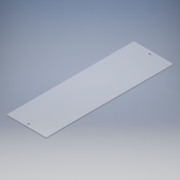
# Autodesk Inventor part: FrontCagePanelRemovable
Saved by Autodesk Inventor 2018 (Build 220112000, 112)
## iProperties
Created: 2013-02-21
Part Number: FrontCagePanelRemovable
Material: PVC-U
Document SubType Name: Modeling
Designer: Neef
Mass: 592.561 g
Surface Area: 1495.34 cm^2
Volume: 423.258 cm^3
Density: 1.29 g/cm^3
Appearance: Smooth - White
Author: Neef
Autodesk Inventor part; units mm, degrees
ref_plane "YZ Plane" through (0, 0, 0) normal (1, 0, 0) x (0, 1, 0)
ref_plane "XZ Plane" through (0, 0, 0) normal (0, 1, 0) x (-1, 0, 0)
ref_plane "XY Plane" through (0, 0, 0) normal (0, 0, 1) x (1, 0, 0)
sketch "Skizze1" plane through (0, 0, 0) normal (0, 0, 1) x (1, 0, 0)
  line L0 (0, 406) -> (0, -406) projected
  line L1 (-126, 0) -> (126, 0) projected
  line L2 (-90, -290) -> (90, -290)
  line L3 (90, -290) -> (90, 290)
  line L4 (90, 290) -> (-90, 290)
  line L5 (-90, 290) -> (-90, -290)
  point P0 (0, 0)
  point P1 (0, -290)
  point P2 (-90, 0)
  dimension "d0" = 580
  dimension "d1" = 180
  constraints: 8 end point, 2 midpoint, 2 parallel, 2 point on line, 1 horizontal, 1 perpendicular
  measures "d0" distance of L4.end L2.start
  measures "d1" distance of L2.start L2.end
extrude "Extrusion1" add sketch "Skizze1" along normal blind 6
sketch "Sketch4" plane through (0, 0, 6) normal (0, 0, 1) x (1, 0, 0)
  circle A0 centre (-3.75, -276) radius 3.825
  line L0 (90, 290) -> (90, -290) projected
  line L1 (90, -290) -> (-90, -290) projected
  circle A1 centre (-3.75, 276) radius 3.825
  line L2 (-90, 290) -> (90, 290) projected
  point P0 (0, 0)
  dimension "d11" = 7.65
  dimension "d12" = 93.75
  dimension "d13" = 14
  dimension "d14" = 7.65
  dimension "d15" = 14
  dimension "d16" = 93.75
  constraints: 2 centre point
  measures "d11" diameter of A0
  measures "d12" distance from line of L0 A0.centre
  measures "d13" distance from line of L1 A0.centre
  measures "d14" diameter of A1
  measures "d15" distance from line of L2 A1.centre
  measures "d16" distance from line of L0 A1.centre
extrude "Extrusion3" cut sketch "Sketch4" against normal blind 10
